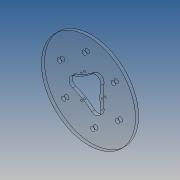
# Autodesk Inventor part: engrane acrílico 2
Saved by Autodesk Inventor 2017 (Build 210142000, 142)
## iProperties
Part Number: engrane acrílico 2
Material: Genérico
Document SubType Name: Modeling
Designer: Leo
Density: 1 g/cm^3
Appearance: Claro - Ligero
Author: Leo
Autodesk Inventor part; units mm, degrees
ref_plane "YZ Plane" through (0, 0, 0) normal (1, 0, 0) x (0, 1, 0)
ref_plane "XZ Plane" through (0, 0, 0) normal (0, 1, 0) x (-1, 0, 0)
ref_plane "XY Plane" through (0, 0, 0) normal (0, 0, 1) x (1, 0, 0)
sketch "Boceto1" plane through (0, 0, 0) normal (0, 1, 0) x (-1, 0, 0)
  circle A0 centre (0, 0) radius 15 construction
  circle A1 centre (0, 0) radius 75
  circle A2 centre (-22, 0) radius 1.5 projected
  circle A3 centre (11, -19.0526) radius 1.5 projected
  circle A4 centre (11, 19.0526) radius 1.5 projected
  arc A5 (25.0049, -8.4836) -> (-5.1555, -25.8966) centre (56.9196, -98.5877) ccw projected
  arc A6 (25.0049, -8.4836) -> (25.0049, 8.4836) centre (22, 0) ccw projected
  arc A7 (-5.1555, 25.8966) -> (25.0049, 8.4836) centre (56.9196, 98.5877) ccw projected
  arc A8 (-5.1555, 25.8966) -> (-19.8494, 17.4131) centre (-11, 19.0526) ccw projected
  arc A9 (-19.8494, -17.4131) -> (-19.8494, 17.4131) centre (-113.8393, 0) ccw projected
  arc A10 (-19.8494, -17.4131) -> (-5.1555, -25.8966) centre (-11, -19.0526) ccw projected
  circle A11 centre (0, 0) radius 15.25 projected
  dimension "d0" = 30
  dimension "d1" = 150
  constraints: 2 centre point, 2 coincident
  measures "d0" diameter of A0
  measures "d1" diameter of A1
extrude "Extrusión2" add sketch "Boceto1" along normal blind 5 contours A1
sketch "Boceto2" plane through (0, 0, 0) normal (0, -1, 0) x (1, 0, 0)
  circle A0 centre (47.4136, -15.577) radius 2.65 construction
  circle A1 centre (47.4136, -15.577) radius 3.5
  circle A2 centre (37.1969, 33.2729) radius 3.5
  circle A3 centre (-10.2168, 48.8499) radius 3.5
  circle A4 centre (-47.4136, 15.577) radius 3.5
  circle A5 centre (-37.1969, -33.2729) radius 3.5
  circle A6 centre (10.2168, -48.8499) radius 3.5
  point P0 (0, 0)
  dimension "d6" = 7
  dimension "d9" = 360
  constraints: 6 centre point, 1 coincident, 13 other
  measures "d6" diameter of A1
extrude "Extrusión3" cut sketch "Boceto2" against normal through all
